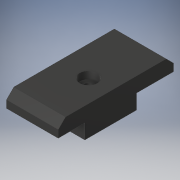
# Autodesk Inventor part: Holding_Plate_Frame
Saved by Autodesk Inventor 2019 (Build 230136000, 136)
## iProperties
Created: 2021-11-06
Part Number: Holding_Plate_Frame
Material: PC/ABS-Kunststoff
Document SubType Name: Modeling
Designer: Bergi
Density: 0.357273 g/cm^3
Appearance: Glatt - Schwarz
Mass: 13.7766 g
Surface Area: 95.3469 cm^2
Volume: 38.5604 cm^3
Author: Bergi
Autodesk Inventor part; units mm, degrees
ref_plane "YZ Plane" through (0, 0, 0) normal (1, 0, 0) x (0, 1, 0)
ref_plane "XZ Plane" through (0, 0, 0) normal (0, 1, 0) x (-1, 0, 0)
ref_plane "XY Plane" through (0, 0, 0) normal (0, 0, 1) x (1, 0, 0)
sketch "Skizze1" plane through (0, 0, 0) normal (0, 1, 0) x (-1, 0, 0)
  line L0 (-17.5, 39) -> (17.5, 39)
  line L1 (17.5, 39) -> (17.5, -39)
  line L2 (17.5, -39) -> (-17.5, -39)
  line L3 (-17.5, -39) -> (-17.5, 39)
  line L4 (-17.5, 39) -> (17.5, -39) construction
  line L5 (17.5, 39) -> (-17.5, -39) construction
  point P0 (0, 0)
  dimension "d0" = 78
  dimension "d1" = 35
  constraints: 12 end point, 2 midpoint, 2 parallel, 1 horizontal, 1 perpendicular
  measures "d0" distance of L0.end L1.end
  measures "d1" distance of L0.start L0.end
extrude "Extrusion1" add sketch "Skizze1" along normal blind 10
sketch "Skizze2" plane through (0, 0, 0) normal (0, -1, 0) x (1, 0, 0)
  line L0 (17.5, 39) -> (-17.5, 39) projected
  line L1 (-17.5, 39) -> (-17.5, -39) projected
  line L2 (-17.5, -39) -> (17.5, -39) projected
  line L3 (17.5, -39) -> (17.5, 39) projected
  line L4 (17.5, 39) -> (17.5, -39) projected
  line L5 (-17.5, -14) -> (17.5, -14)
  line L6 (17.5, -14) -> (17.5, 21)
  line L7 (17.5, 21) -> (-17.5, 21)
  line L8 (-17.5, 21) -> (-17.5, -14)
  point P0 (0, 0)
  dimension "d4" = 18
  dimension "d5" = 25
  constraints: 8 end point, 2 parallel, 2 point on line, 1 horizontal, 1 perpendicular
  measures "d4" distance between parallel lines of L0 L7
  measures "d5" distance between parallel lines of L5 L2
extrude "Extrusion2" add sketch "Skizze2" along normal blind 10 contours L3 L5 L1 L7
sketch "Skizze3" plane through (0, 10, 0) normal (0, 1, 0) x (1, 0, 0)
  line L0 (17.5, -39) -> (17.5, 39) projected
  line L1 (-17.5, -39) -> (17.5, -39) projected
  point P0 (0, 0)
  point P1 (2.5, -3.5)
  dimension "d8" = 15
  dimension "d9" = 35.5
  measures "d8" distance from line of L0 point (2.5, -3.5)
  measures "d9" distance from line of L1 point (2.5, -3.5)
hole "Bohrung1" at (2.5, 10, 3.5) direction (0, -1, 0) diameter 6 end through all counterbore diameter 12 counterbore depth 5
chamfer "Fase1" distance 5 angle 45 2 edges at (0, 10, 39) (0, 10, -39)
